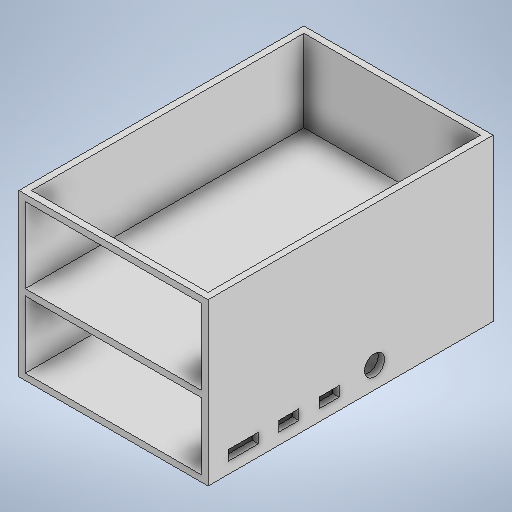
# Autodesk Inventor part: Pi_FPGA_Board_Case
Saved by Autodesk Inventor 2025 (Build 290162000, 162)
## iProperties
Created: 2024-06-19
Part Number: Pi_FPGA_Board_Case
Material: Generic
Document SubType Name: Modeling
Designer: track
Density: 1 g/cm^3
Appearance: Default
Author: track
Autodesk Inventor part; units mm, degrees
ref_plane "YZ Plane" through (0, 0, 0) normal (1, 0, 0) x (0, 1, 0)
ref_plane "XZ Plane" through (0, 0, 0) normal (0, 1, 0) x (-1, 0, 0)
ref_plane "XY Plane" through (0, 0, 0) normal (0, 0, 1) x (1, 0, 0)
sketch "Sketch1" plane through (0, 0, 0) normal (0, 1, 0) x (-1, 0, 0)
  line L0 (-27.7812, -42.8625) -> (27.7813, -42.8625)
  line L1 (27.7813, -42.8625) -> (27.7812, 42.8625)
  line L2 (27.7812, 42.8625) -> (-27.7813, 42.8625)
  line L3 (-27.7813, 42.8625) -> (-27.7812, -42.8625)
  line L4 (-27.7812, -42.8625) -> (27.7812, 42.8625) construction
  line L5 (27.7813, -42.8625) -> (-27.7813, 42.8625) construction
  line L6 (-29.7812, -44.8625) -> (29.7813, -44.8625)
  line L7 (29.7813, -44.8625) -> (29.7812, 44.8625)
  line L8 (29.7812, 44.8625) -> (-29.7813, 44.8625)
  line L9 (-29.7813, 44.8625) -> (-29.7812, -44.8625)
  point P0 (0, 0)
  dimension "d0" = 85.725
  dimension "d1" = 55.5625
  dimension "d2" = 2
  constraints: 20 end point, 4 parallel, 2 midpoint, 2 perpendicular, 1 horizontal, 3 other
  measures "d0" distance of L0.end L1.end
  measures "d1" distance of L0.start L0.end
  measures "d2" distance between parallel lines of L6 L0
extrude "Extrusion1" add sketch "Sketch1" along normal blind 50.8
sketch "Sketch2" plane through (0, 0, 0) normal (0, 1, 0) x (-1, 0, 0)
  line L0 (27.7812, 42.8625) -> (27.7813, -42.8625) projected
  line L1 (-27.7813, 42.8625) -> (27.7813, 42.8625)
  line L2 (27.7813, 42.8625) -> (27.7813, -42.8625)
  line L3 (27.7813, -42.8625) -> (-27.7813, -42.8625)
  line L4 (-27.7813, -42.8625) -> (-27.7813, 42.8625)
  line L5 (-27.7813, 42.8625) -> (27.7813, -42.8625) construction
  line L6 (27.7813, 42.8625) -> (-27.7813, -42.8625) construction
  point P0 (0, 0)
  constraints: 12 end point, 2 midpoint, 2 parallel, 1 horizontal, 1 perpendicular
extrude "Extrusion2" add sketch "Sketch2" along normal blind 2
sketch "Sketch3" plane through (-29.7812, 0, 44.8625) normal (0, 0, 1) x (1, 0, 0)
  line L0 (59.5625, 50.8) -> (0, 50.8) projected
  line L1 (59.5625, 0) -> (0, 0) projected
  line L2 (0, 50.8) -> (59.5625, 50.8)
  line L3 (59.5625, 50.8) -> (59.5625, 0)
  line L4 (59.5625, 0) -> (0, 0)
  line L5 (0, 0) -> (0, 50.8)
  line L6 (57.5625, 2) -> (57.5625, 48.8)
  line L7 (57.5625, 48.8) -> (2, 48.8)
  line L8 (2, 48.8) -> (2, 2)
  line L9 (2, 2) -> (57.5625, 2)
  dimension "d12" = 2
  constraints: 16 end point, 4 parallel, 2 perpendicular, 1 horizontal, 3 other
  measures "d12" distance between parallel lines of L3 L6
extrude "Extrusion3" cut sketch "Sketch3" against normal up to surface (2 mm away) contours L9 L8 L7 L6
sketch "Sketch4" plane through (-27.7813, 50.8, -42.8625) normal (0, 0, 1) x (1, 0, 0)
  line L0 (1.5875, -47.2125) -> (17.4625, -47.2125)
  line L1 (17.4625, -47.2125) -> (17.4625, -34.5125)
  line L2 (17.4625, -34.5125) -> (1.5875, -34.5125)
  line L3 (1.5875, -34.5125) -> (1.5875, -47.2125)
  line L4 (22.225, -47.2125) -> (34.925, -47.2125)
  line L5 (34.925, -47.2125) -> (34.925, -29.75)
  line L6 (34.925, -29.75) -> (22.225, -29.75)
  line L7 (22.225, -29.75) -> (22.225, -47.2125)
  line L8 (0, -48.8) -> (0, -2) projected
  line L9 (55.5625, -48.8) -> (0, -48.8) projected
  line L10 (39.6875, -47.2125) -> (52.3875, -47.2125)
  line L11 (52.3875, -47.2125) -> (52.3875, -29.75)
  line L12 (52.3875, -29.75) -> (39.6875, -29.75)
  line L13 (39.6875, -29.75) -> (39.6875, -47.2125)
  point P0 (27.7813, -50.8)
  dimension "d17" = 1.5875
  dimension "d18" = 1.5875
  dimension "d20" = 19.05
  dimension "d21" = 1.5875
  dimension "d22" = 4.7625
  dimension "d23" = 4.7625
  dimension "d24" = 12.7
  dimension "d30" = 14.2875
  dimension "d31" = 19.05
  dimension "d32" = 1.5875
  dimension "d33" = 15.875
  dimension "d34" = 12.7
  constraints: 24 end point, 6 parallel, 3 horizontal, 3 perpendicular, 1 point on line
  measures "d17" distance between parallel lines of L9 L0
  measures "d18" distance between parallel lines of L9 L4
  measures "d20" distance between parallel lines of L9 L6
  measures "d21" distance between parallel lines of L9 L10
  measures "d22" distance between parallel lines of L1 L7
  measures "d23" distance between parallel lines of L13 L5
  measures "d24" distance of L5.end L6.end
  measures "d30" distance between parallel lines of L9 L2
  measures "d31" distance between parallel lines of L9 L12
  measures "d32" distance between parallel lines of L8 L3
  measures "d33" distance of L1.end L2.end
  measures "d34" distance of L11.end L12.end
extrude "Extrusion4" cut sketch "Sketch4" against normal up to surface (2 mm away)
sketch "Sketch5" plane through (-27.7813, 50.8, -42.8625) normal (0, 0, 1) x (1, 0, 0)
  line L0 (55.5625, -48.8) -> (55.5625, 0) projected
  line L1 (0, -48.8) -> (0, 0) projected
  line L2 (55.5625, -27.75) -> (0, -27.75)
  line L3 (0, -27.75) -> (0, -25.75)
  line L4 (0, -25.75) -> (55.5625, -25.75)
  line L5 (55.5625, -25.75) -> (55.5625, -27.75)
  line L6 (39.6875, -29.75) -> (52.3875, -29.75) projected
  point P0 (27.7813, -50.8)
  point P1 (0, -27.75)
  dimension "d35" = 2
  dimension "d36" = 2
  constraints: 8 end point, 2 parallel, 2 point on line, 1 horizontal, 1 perpendicular
  measures "d35" distance between parallel lines of L2 L6
  measures "d36" distance between parallel lines of L2 L4
extrude "Extrusion5" add sketch "Sketch5" along normal up to surface (87.725 mm away)
sketch "Sketch6" plane through (29.7813, 0, 44.8625) normal (1, 0, 0) x (0, 0, -1)
  line L0 (89.725, 23.05) -> (0, 23.05)
  line L1 (0, 23.05) -> (0, 2)
  line L2 (0, 0) -> (0, 50.8) projected
  line L3 (0, 2) -> (89.725, 2)
  line L4 (89.725, 21.05) -> (89.725, 3.5875) projected
  line L5 (89.725, 23.05) -> (89.725, 2)
  line L6 (89.725, 0) -> (89.725, 50.8) projected
  line L7 (0, 0) -> (89.725, 0) projected
  line L8 (6.35, 6.7625) -> (15.875, 6.7625)
  line L9 (15.875, 6.7625) -> (15.875, 3.5875)
  line L10 (15.875, 3.5875) -> (6.35, 3.5875)
  line L11 (6.35, 3.5875) -> (6.35, 6.7625)
  line L12 (22.225, 6.7625) -> (28.575, 6.7625)
  line L13 (28.575, 6.7625) -> (28.575, 3.5875)
  line L14 (28.575, 3.5875) -> (22.225, 3.5875)
  line L15 (22.225, 3.5875) -> (22.225, 6.7625)
  line L16 (34.925, 6.7625) -> (41.275, 6.7625)
  line L17 (41.275, 6.7625) -> (41.275, 3.5875)
  line L18 (41.275, 3.5875) -> (34.925, 3.5875)
  line L19 (34.925, 3.5875) -> (34.925, 6.7625)
  circle A0 centre (52.3875, 6.7625) radius 3.175
  point P0 (44.8625, 0)
  dimension "d40" = 0
  dimension "d41" = 2
  dimension "d42" = 89.725
  dimension "d43" = 90
  dimension "d44" = 6.35
  dimension "d45" = 9.525
  dimension "d46" = 1.5875
  dimension "d47" = 3.175
  dimension "d48" = 15.875
  dimension "d49" = 1.5875
  dimension "d50" = 1.5875
  dimension "d51" = 6.35
  dimension "d52" = 4.7625
  dimension "d53" = 12.7
  dimension "d54" = 3.175
  dimension "d55" = 3.175
  dimension "d56" = 6.35
  dimension "d57" = 6.35
  dimension "d58" = 11.1125
  constraints: 32 end point, 6 parallel, 4 horizontal, 3 perpendicular, 2 point on line, 1 centre point, 1 collinear
  measures "d40" distance from line of L1.start L0
  measures "d41" distance between parallel lines of L7 L3
  measures "d42" distance of L0.start L0.end
  measures "d43" angle of L0 L1
  measures "d44" distance between parallel lines of L1 L11
  measures "d45" distance of L8.start L8.end
  measures "d46" distance between parallel lines of L3 L10
  measures "d47" distance between parallel lines of L8 L10
  measures "d48" distance between parallel lines of L15 L11
  measures "d49" distance between parallel lines of L3 L14
  measures "d50" distance between parallel lines of L3 L18
  measures "d51" diameter of A0
  measures "d52" distance from line of L3 A0.centre
  measures "d53" distance between parallel lines of L19 L15
  measures "d54" distance between parallel lines of L14 L12
  measures "d55" distance between parallel lines of L18 L16
  measures "d56" distance of L12.start L12.end
  measures "d57" distance of L16.start L16.end
  measures "d58" distance from line of A0.centre L17
extrude "Extrusion6" cut sketch "Sketch6" against normal up to surface (2 mm away) contours L8 L9 L10 L11 | L12 L13 L14 L15 | L16 L17 L18 L19 | A0
body "Solid1"
